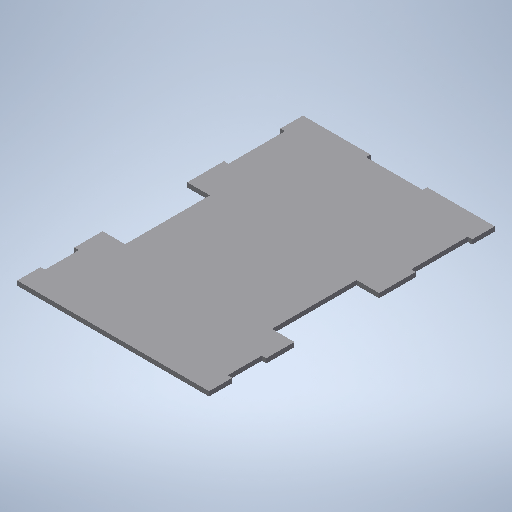
# Autodesk Inventor part: Parte inf
Saved by Autodesk Inventor 2025 (Build 290162000, 162)
## iProperties
Created: 2024-10-07
Part Number: Parte inf
Material: Generic
Document SubType Name: Modeling
Designer: feder
Density: 1 g/cm^3
Appearance: Default
Author: feder
Autodesk Inventor part; units mm, degrees
ref_plane "YZ Plane" through (0, 0, 0) normal (1, 0, 0) x (0, 1, 0)
ref_plane "XZ Plane" through (0, 0, 0) normal (0, 1, 0) x (-1, 0, 0)
ref_plane "XY Plane" through (0, 0, 0) normal (0, 0, 1) x (1, 0, 0)
sketch "Sketch1" plane through (0, 0, 0) normal (0, 1, 0) x (-1, 0, 0)
  line L0 (85, 100) -> (-85, 100)
  line L1 (-85, 100) -> (-85, -100)
  line L2 (-85, -100) -> (85, -100)
  line L3 (85, -100) -> (85, 100)
  point P0 (0, 0)
  point P1 (0, -100)
  dimension "d0" = 200
  dimension "d1" = 170
  dimension "d15" = 100
  dimension "d16" = 0
  constraints: 8 end point, 2 parallel, 1 horizontal, 1 midpoint, 1 perpendicular
  measures "d0" distance of L2.end L0.start
  measures "d1" distance of L1.end L2.end
  measures "d15" distance of point (0, 0) point (0, -100)
  measures "d16" horizontal distance of point (0, 0) point (0, -100)
extrude "Extrusion1" add sketch "Sketch1" along normal blind 4
sketch "Sketch2" plane through (85, 0, -100) normal (0, 0, -1) x (-1, 0, 0)
  line L0 (0, 4) -> (169.1447, 65.5636)
  line L1 (0, 4) -> (-1.7101, 8.6985)
  line L2 (-1.7101, 8.6985) -> (167.4346, 70.2621)
  line L3 (167.4346, 70.2621) -> (169.1447, 65.5636)
  line L4 (0, 4) -> (-10.9899, 0)
  line L5 (0, 0) -> (170, 0) projected
  line L6 (-10.9899, 0) -> (-12.7, 4.6985)
  line L7 (-12.7, 4.6985) -> (-1.7101, 8.6985)
  point P0 (85, 0)
  dimension "d4" = 180
  dimension "d5" = 5
  dimension "d6" = 20
  dimension "d7" = 20
  constraints: 14 end point, 3 perpendicular, 1 collinear, 1 point on line
  measures "d4" distance of L0.start L0.end
  measures "d5" distance of L0.start L1.end
  measures "d6" angle of L5 L0
  measures "d7" angle of L5 L2
extrude "Extrusion2" [suppressed]
sketch "Sketch3" plane through (0, 0, 0) normal (0, -1, 0) x (1, 0, 0)
  line L0 (-85, -100) -> (-85, 100) projected
  line L1 (-85, 77.5) -> (-65, 77.5)
  line L2 (-65, 77.5) -> (-65, 2.5)
  line L3 (-65, 2.5) -> (-85, 2.5)
  line L4 (-85, 2.5) -> (-85, 77.5)
  point P0 (0, 0)
  point P1 (-65, 40)
  dimension "d10" = 20
  dimension "d11" = 75
  dimension "d12" = 40
  constraints: 8 end point, 2 parallel, 1 horizontal, 1 midpoint, 1 perpendicular, 1 point on line
  measures "d10" distance of L1.start L1.end
  measures "d11" distance of L1.end L2.end
  measures "d12" vertical distance of point (0, 0) point (-65, 40)
extrude "Extrusion3" cut sketch "Sketch3" against normal through all
mirror "Mirror1" about plane through (0, 0, 0) normal (1, 0, 0) of "Extrusion3"
sketch "Sketch4" plane through (0, 4, 0) normal (0, 1, 0) x (1, 0, 0)
  line L0 (25, 100) -> (-25, 100)
  line L1 (-25, 100) -> (-25, 96)
  line L2 (-25, 96) -> (25, 96)
  line L3 (25, 96) -> (25, 100)
  point P0 (0, 0)
  point P1 (0, 96)
  dimension "d17" = 4
  dimension "d18" = 96
  dimension "d19" = 50
  constraints: 8 end point, 2 parallel, 1 horizontal, 1 midpoint, 1 perpendicular, 1 vertical alignment
  measures "d17" distance of L2.end L0.start
  measures "d18" distance of point (0, 0) point (0, 96)
  measures "d19" distance of L1.end L2.end
extrude "Extrusion4" cut sketch "Sketch4" against normal through all
sketch "Sketch5" plane through (0, 4, 0) normal (0, 1, 0) x (1, 0, 0)
  line L0 (-85, 100) -> (-85, -2.5) projected
  line L1 (-85, 80) -> (-81, 80)
  line L2 (-81, 80) -> (-81, 30)
  line L3 (-81, 30) -> (-85, 30)
  line L4 (-85, 30) -> (-85, 80)
  line L5 (-85, -100) -> (85, -100) projected
  point P0 (0, 0)
  dimension "d22" = 50
  dimension "d23" = 4
  dimension "d24" = 20
  constraints: 8 end point, 2 parallel, 1 horizontal, 1 perpendicular, 1 point on line
  measures "d22" distance of L1.end L2.end
  measures "d23" distance of L2.end L3.end
  measures "d24" distance from line of L1 L0.start
extrude "Extrusion5" cut sketch "Sketch5" against normal through all
mirror "Mirror2" about plane through (0, 0, 0) normal (1, 0, 0) of "Extrusion5"
sketch "Sketch6" plane through (-85, 0, 100) normal (0, 0, 1) x (1, 0, 0)
  line L0 (150, 4) -> (170, 4) projected
  line L1 (0, 0) -> (170, 0)
  line L2 (170, 0) -> (170, 4)
  line L3 (170, 4) -> (0, 4)
  line L4 (0, 4) -> (0, 0)
  point P0 (85, 0)
  constraints: 8 end point, 2 parallel, 1 horizontal, 1 perpendicular
extrude "Extrusion6" add sketch "Sketch6" along normal blind 53.169
sketch "Sketch7" plane through (0, 4, 0) normal (0, 1, 0) x (1, 0, 0)
  line L0 (-85, -77.5) -> (-85, -153.169) projected
  line L1 (-85, -102.5) -> (-81, -102.5)
  line L2 (-81, -102.5) -> (-81, -132.5)
  line L3 (-81, -132.5) -> (-85, -132.5)
  line L4 (-85, -132.5) -> (-85, -102.5)
  line L5 (-65, -77.5) -> (-85, -77.5) projected
  point P0 (0, 0)
  point P1 (-83, -102.5)
  dimension "d32" = 30
  dimension "d33" = 4
  dimension "d34" = 25
  constraints: 8 end point, 2 parallel, 1 horizontal, 1 midpoint, 1 perpendicular, 1 point on line
  measures "d32" distance of L1.end L2.end
  measures "d33" distance of L2.end L3.end
  measures "d34" distance from line of point (-83, -102.5) L5
extrude "Extrusion7" cut sketch "Sketch7" against normal blind 10
mirror "Mirror3" about plane through (0, 0, 0) normal (1, 0, 0) of "Extrusion7"
body "Solid1"
